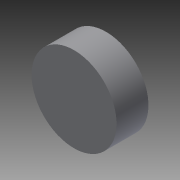
# Autodesk Inventor part: Wheel_cap
Saved by Autodesk Inventor 2015 (Build 190159000, 159)
## iProperties
Created: 2014-11-06
Part Number: Wheel_cap
Material: Generic
Document SubType Name: Modeling
Designer: bpowe_000
Density: 1 g/cm^3
Appearance: Default
Author: bpowe_000
Autodesk Inventor part; units mm, degrees
ref_plane "YZ Plane" through (0, 0, 0) normal (1, 0, 0) x (0, 1, 0)
ref_plane "XZ Plane" through (0, 0, 0) normal (0, 1, 0) x (-1, 0, 0)
ref_plane "XY Plane" through (0, 0, 0) normal (0, 0, 1) x (1, 0, 0)
sketch "Sketch1" plane through (0, 0, 0) normal (0, 1, 0) x (-1, 0, 0)
  circle A0 centre (0, 0) radius 4
  dimension "d0" = 8
  constraints: 1 centre point, 1 coincident
  measures "d0" diameter of A0
extrude "Extrusion1" add sketch "Sketch1" along normal blind 3
sketch "Sketch2" plane through (0, 3, 0) normal (0, 1, 0) x (1, 0, 0)
  line L0 (-1.595, -1.595) -> (1.595, -1.595)
  line L1 (1.595, -1.595) -> (1.595, 1.595)
  line L2 (1.595, 1.595) -> (-1.595, 1.595)
  line L3 (-1.595, 1.595) -> (-1.595, -1.595)
  point P0 (0, 0)
  dimension "d3" = 3.19
  dimension "d4" = 1.595
  dimension "d6" = 1.595
  constraints: 8 end point, 2 parallel, 2 perpendicular, 1 horizontal
  measures "d3" distance of L2.end L0.start
  measures "d4" distance from line of L0 point (0, 0)
  measures "d6" distance from line of L1 point (0, 0)
extrude "Extrusion2" cut sketch "Sketch2" against normal blind 1.5
equation "\"d4\" = 0.5 * d3"
equation "\"d6\" = 0.5 * d3"
body "Solid1"
